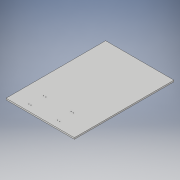
# Autodesk Inventor part: main plate
Saved by Autodesk Inventor 2019 (Build 230136000, 136)
## iProperties
Created: 2020-10-03
Part Number: main plate
Material: Generic
Document SubType Name: Modeling
Designer: User
Density: 1 g/cm^3
Appearance: Default
Author: User
Autodesk Inventor part; units mm, degrees
ref_plane "YZ Plane" through (0, 0, 0) normal (1, 0, 0) x (0, 1, 0)
ref_plane "XZ Plane" through (0, 0, 0) normal (0, 1, 0) x (-1, 0, 0)
ref_plane "XY Plane" through (0, 0, 0) normal (0, 0, 1) x (1, 0, 0)
sketch "Sketch1" plane through (0, 0, 0) normal (0, 1, 0) x (-1, 0, 0)
  line L0 (0, 0) -> (304.8, 0)
  line L1 (304.8, 0) -> (304.8, -444.5)
  line L2 (304.8, -444.5) -> (0, -444.5)
  line L3 (0, -444.5) -> (0, 0)
  dimension "d0" = 304.8
  dimension "d1" = 444.5
  constraints: 8 end point, 2 parallel, 1 horizontal, 1 perpendicular
  measures "d0" distance of L1.end L2.end
  measures "d1" distance of L0.end L1.end
extrude "Extrusion1" add sketch "Sketch1" along normal blind 6.35
sketch "Sketch2" plane through (0, 6.35, 0) normal (0, 1, 0) x (1, 0, 0)
  circle A0 centre (-95.1484, 30.099) radius 1.3589
  circle A1 centre (-105.156, 30.099) radius 1.3589
  line L0 (-304.8, 0) -> (0, 0) projected
  line L1 (0, 0) -> (0, 444.5) projected
  dimension "d4" = 2.7178
  dimension "d5" = 2.7178
  dimension "d7" = 95.1484
  dimension "d8" = 10.0076
  dimension "d9" = 30.099
  dimension "d37" = 30.099
  constraints: 2 centre point
  measures "d4" diameter of A0
  measures "d5" diameter of A1
  measures "d7" distance from line of L1 A0.centre
  measures "d8" distance of A1.centre A0.centre
  measures "d9" distance from line of L0 A1.centre
  measures "d37" distance from line of L0 A0.centre
extrude "Extrusion2" cut sketch "Sketch2" against normal blind 25.4
sketch "Sketch3" plane through (0, 6.35, 0) normal (0, 1, 0) x (1, 0, 0)
  circle A0 centre (-107.696, 93.1418) radius 1.3589
  circle A1 centre (-97.6884, 93.1418) radius 1.3589
  circle A2 centre (-95.1484, 30.099) radius 1.3589 projected
  circle A3 centre (-105.156, 30.099) radius 1.3589 projected
  line L0 (0, 0) -> (0, 444.5) projected
  dimension "d12" = 2.7178
  dimension "d13" = 2.7178
  dimension "d14" = 63.0428
  dimension "d15" = 63.0428
  dimension "d16" = 10.0076
  dimension "d17" = 97.6884
  constraints: 2 centre point
  measures "d12" diameter of A0
  measures "d13" diameter of A1
  measures "d14" vertical distance of A1.centre A2.centre
  measures "d15" vertical distance of A3.centre A0.centre
  measures "d16" distance of A0.centre A1.centre
  measures "d17" distance from line of L0 A1.centre
extrude "Extrusion3" cut sketch "Sketch3" against normal blind 25.4 contours A0 | A1
sketch "Sketch4" plane through (0, 6.35, 0) normal (0, 1, 0) x (1, 0, 0)
  circle A0 centre (-230.4034, 93.091) radius 1.3589
  circle A1 centre (-220.3962, 93.1789) radius 1.3589
  line L0 (-304.8, 444.5) -> (-304.8, 0) projected
  line L1 (-304.8, 0) -> (0, 0) projected
  dimension "d20" = 2.7178
  dimension "d21" = 2.7178
  dimension "d22" = 10.0076
  dimension "d23" = 74.3966
  dimension "d24" = 93.091
  constraints: 2 centre point
  measures "d20" diameter of A0
  measures "d21" diameter of A1
  measures "d22" distance of A1.centre A0.centre
  measures "d23" distance from line of L0 A0.centre
  measures "d24" distance from line of L1 A0.centre
extrude "Extrusion4" cut sketch "Sketch4" against normal blind 25.4
sketch "Sketch5" plane through (0, 6.35, 0) normal (0, 1, 0) x (1, 0, 0)
  circle A0 centre (-232.029, 28.702) radius 1.3589
  circle A1 centre (-222.0214, 28.702) radius 1.3589
  line L0 (-304.8, 0) -> (0, 0) projected
  line L1 (-304.8, 444.5) -> (-304.8, 0) projected
  line L2 (0, 0) -> (0, 444.5) projected
  dimension "d27" = 2.7178
  dimension "d28" = 2.7178
  dimension "d31" = 28.702
  dimension "d32" = 10.0076
  dimension "d36" = 222.0214
  dimension "d38" = 28.702
  constraints: 2 centre point
  measures "d27" diameter of A0
  measures "d28" diameter of A1
  measures "d31" distance from line of L0 A0.centre
  measures "d32" distance of A1.centre A0.centre
  measures "d36" distance from line of L2 A1.centre
  measures "d38" distance from line of L0 A1.centre
extrude "Extrusion5" cut sketch "Sketch5" against normal blind 25.4
body "Solid1"
